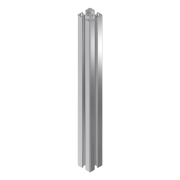
# Autodesk Inventor part: Propile_355
Saved by Autodesk Inventor 2019 (Build 230136000, 136)
## iProperties
Created: 2019-04-24
Part Number: Propile_355
Material: 알루미늄 6061
Document SubType Name: Modeling
Designer: hinmo
Mass: 308.007 g
Surface Area: 1319.64 cm^2
Volume: 114.076 cm^3
Density: 2.7 g/cm^3
Appearance: 알루미늄 - 평지
Author: hinmo
Autodesk Inventor part; units mm, degrees
ref_plane "YZ Plane" through (0, 0, 0) normal (1, 0, 0) x (0, 1, 0)
ref_plane "XZ Plane" through (0, 0, 0) normal (0, 1, 0) x (-1, 0, 0)
ref_plane "XY Plane" through (0, 0, 0) normal (0, 0, 1) x (1, 0, 0)
sketch "스케치1" plane through (0, 0, 0) normal (0, 1, 0) x (-1, 0, 0)
  arc A0 (-198.9025, -155.31) -> (-197.9025, -154.31) centre (-198.9025, -154.31) ccw projected
  line L0 (-197.9025, -154.31) -> (-197.9025, -152.81) projected
  line L1 (-197.9025, -152.81) -> (-199.8525, -152.81) projected
  line L2 (-199.8525, -152.81) -> (-200.8313, -149.1169) projected
  arc A1 (-198.1875, -144.81) -> (-200.8313, -149.1169) centre (-194.1553, -150.25) ccw projected
  line L3 (-198.1875, -144.81) -> (-195.2525, -144.81) projected
  line L4 (-195.2525, -144.81) -> (-194.7525, -144.31) projected
  line L5 (-194.7525, -144.31) -> (-194.2525, -144.81) projected
  line L6 (-194.2525, -144.81) -> (-191.3175, -144.81) projected
  arc A2 (-188.6738, -149.1169) -> (-191.3175, -144.81) centre (-195.3497, -150.25) ccw projected
  line L7 (-188.6738, -149.1169) -> (-189.6525, -152.81) projected
  line L8 (-189.6525, -152.81) -> (-191.6025, -152.81) projected
  line L9 (-191.6025, -152.81) -> (-191.6025, -154.31) projected
  arc A3 (-191.6025, -154.31) -> (-190.6025, -155.31) centre (-190.6025, -154.31) ccw projected
  line L10 (-190.6025, -155.31) -> (-181.2525, -155.31) projected
  arc A4 (-181.2525, -155.31) -> (-179.7525, -153.81) centre (-181.2525, -153.81) ccw projected
  line L11 (-179.7525, -153.81) -> (-179.7525, -144.46) projected
  arc A5 (-179.7525, -144.46) -> (-180.7525, -143.46) centre (-180.7525, -144.46) ccw projected
  line L12 (-180.7525, -143.46) -> (-182.2525, -143.46) projected
  line L13 (-182.2525, -143.46) -> (-182.2525, -145.41) projected
  line L14 (-182.2525, -145.41) -> (-185.9457, -146.3887) projected
  arc A6 (-190.2525, -143.745) -> (-185.9457, -146.3887) centre (-184.8126, -139.7128) ccw projected
  line L15 (-190.2525, -143.745) -> (-190.2525, -140.81) projected
  line L16 (-190.2525, -140.81) -> (-190.7525, -140.31) projected
  line L17 (-190.7525, -140.31) -> (-190.2525, -139.81) projected
  line L18 (-190.2525, -139.81) -> (-190.2525, -136.875) projected
  arc A7 (-185.9457, -134.2313) -> (-190.2525, -136.875) centre (-184.8126, -140.9072) ccw projected
  line L19 (-185.9457, -134.2313) -> (-182.2525, -135.21) projected
  line L20 (-182.2525, -135.21) -> (-182.2525, -137.16) projected
  line L21 (-182.2525, -137.16) -> (-180.7525, -137.16) projected
  arc A8 (-180.7525, -137.16) -> (-179.7525, -136.16) centre (-180.7525, -136.16) ccw projected
  line L22 (-179.7525, -136.16) -> (-179.7525, -126.81) projected
  arc A9 (-179.7525, -126.81) -> (-181.2525, -125.31) centre (-181.2525, -126.81) ccw projected
  line L23 (-181.2525, -125.31) -> (-190.6025, -125.31) projected
  arc A10 (-190.6025, -125.31) -> (-191.6025, -126.31) centre (-190.6025, -126.31) ccw projected
  line L24 (-191.6025, -126.31) -> (-191.6025, -127.81) projected
  line L25 (-191.6025, -127.81) -> (-189.6525, -127.81) projected
  line L26 (-189.6525, -127.81) -> (-188.6738, -131.5032) projected
  arc A11 (-191.3175, -135.81) -> (-188.6738, -131.5032) centre (-195.3497, -130.37) ccw projected
  line L27 (-191.3175, -135.81) -> (-194.2525, -135.81) projected
  line L28 (-194.2525, -135.81) -> (-194.7525, -136.31) projected
  line L29 (-194.7525, -136.31) -> (-195.2525, -135.81) projected
  line L30 (-195.2525, -135.81) -> (-198.1875, -135.81) projected
  arc A12 (-200.8313, -131.5032) -> (-198.1875, -135.81) centre (-194.1553, -130.37) ccw projected
  line L31 (-200.8313, -131.5032) -> (-199.8525, -127.81) projected
  line L32 (-199.8525, -127.81) -> (-197.9025, -127.81) projected
  line L33 (-197.9025, -127.81) -> (-197.9025, -126.31) projected
  arc A13 (-197.9025, -126.31) -> (-198.9025, -125.31) centre (-198.9025, -126.31) ccw projected
  line L34 (-198.9025, -125.31) -> (-208.2525, -125.31) projected
  arc A14 (-208.2525, -125.31) -> (-209.7525, -126.81) centre (-208.2525, -126.81) ccw projected
  line L35 (-209.7525, -126.81) -> (-209.7525, -136.16) projected
  arc A15 (-209.7525, -136.16) -> (-208.7525, -137.16) centre (-208.7525, -136.16) ccw projected
  line L36 (-208.7525, -137.16) -> (-207.2525, -137.16) projected
  line L37 (-207.2525, -137.16) -> (-207.2525, -135.21) projected
  line L38 (-207.2525, -135.21) -> (-203.5594, -134.2313) projected
  arc A16 (-199.2525, -136.875) -> (-203.5594, -134.2313) centre (-204.6925, -140.9072) ccw projected
  line L39 (-199.2525, -136.875) -> (-199.2525, -139.81) projected
  line L40 (-199.2525, -139.81) -> (-198.7525, -140.31) projected
  line L41 (-198.7525, -140.31) -> (-199.2525, -140.81) projected
  line L42 (-199.2525, -140.81) -> (-199.2525, -143.745) projected
  arc A17 (-203.5594, -146.3887) -> (-199.2525, -143.745) centre (-204.6925, -139.7128) ccw projected
  line L43 (-203.5594, -146.3887) -> (-207.2525, -145.41) projected
  line L44 (-207.2525, -145.41) -> (-207.2525, -143.46) projected
  line L45 (-207.2525, -143.46) -> (-208.7525, -143.46) projected
  arc A18 (-208.7525, -143.46) -> (-209.7525, -144.46) centre (-208.7525, -144.46) ccw projected
  line L46 (-209.7525, -144.46) -> (-209.7525, -153.81) projected
  arc A19 (-209.7525, -153.81) -> (-208.2525, -155.31) centre (-208.2525, -153.81) ccw projected
  line L47 (-208.2525, -155.31) -> (-198.9025, -155.31) projected
  arc A20 (-182.1682, -131.8336) -> (-182.1682, -128.7864) centre (-184.7525, -130.31) ccw projected
  line L48 (-182.1682, -131.8336) -> (-181.2222, -132.7797) projected
  line L49 (-181.2222, -132.7797) -> (-182.2829, -133.8403) projected
  line L50 (-182.2829, -133.8403) -> (-183.2289, -132.8943) projected
  arc A21 (-186.2762, -132.8943) -> (-183.2289, -132.8943) centre (-184.7525, -130.31) ccw projected
  line L51 (-186.2762, -132.8943) -> (-187.2222, -133.8403) projected
  line L52 (-187.2222, -133.8403) -> (-188.2829, -132.7797) projected
  line L53 (-188.2829, -132.7797) -> (-187.3368, -131.8336) projected
  arc A22 (-187.3368, -128.7864) -> (-187.3368, -131.8336) centre (-184.7525, -130.31) ccw projected
  line L54 (-187.3368, -128.7864) -> (-188.2829, -127.8403) projected
  line L55 (-188.2829, -127.8403) -> (-187.2222, -126.7797) projected
  line L56 (-187.2222, -126.7797) -> (-186.2762, -127.7257) projected
  arc A23 (-183.2289, -127.7257) -> (-186.2762, -127.7257) centre (-184.7525, -130.31) ccw projected
  line L57 (-183.2289, -127.7257) -> (-182.2829, -126.7797) projected
  line L58 (-182.2829, -126.7797) -> (-181.2222, -127.8403) projected
  line L59 (-181.2222, -127.8403) -> (-182.1682, -128.7864) projected
  line L60 (-191.7222, -138.3403) -> (-192.6564, -138.9476) projected
  arc A24 (-192.6564, -141.6725) -> (-192.6564, -138.9476) centre (-194.7525, -140.31) ccw projected
  line L61 (-192.6564, -141.6725) -> (-191.7222, -142.2797) projected
  line L62 (-191.7222, -142.2797) -> (-192.7829, -143.3403) projected
  line L63 (-192.7829, -143.3403) -> (-193.3901, -142.4061) projected
  arc A25 (-196.115, -142.4061) -> (-193.3901, -142.4061) centre (-194.7525, -140.31) ccw projected
  line L64 (-196.115, -142.4061) -> (-196.7222, -143.3403) projected
  line L65 (-196.7222, -143.3403) -> (-197.7829, -142.2797) projected
  line L66 (-197.7829, -142.2797) -> (-196.8487, -141.6725) projected
  arc A26 (-196.8487, -138.9476) -> (-196.8487, -141.6725) centre (-194.7525, -140.31) ccw projected
  line L67 (-196.8487, -138.9476) -> (-197.7829, -138.3403) projected
  line L68 (-197.7829, -138.3403) -> (-196.7222, -137.2797) projected
  line L69 (-196.7222, -137.2797) -> (-196.115, -138.2139) projected
  arc A27 (-193.3901, -138.2139) -> (-196.115, -138.2139) centre (-194.7525, -140.31) ccw projected
  line L70 (-193.3901, -138.2139) -> (-192.7829, -137.2797) projected
  line L71 (-192.7829, -137.2797) -> (-191.7222, -138.3403) projected
  arc A28 (-183.2289, -147.7257) -> (-186.2762, -147.7257) centre (-184.7525, -150.31) ccw projected
  line L72 (-183.2289, -147.7257) -> (-182.2829, -146.7797) projected
  line L73 (-182.2829, -146.7797) -> (-181.2222, -147.8403) projected
  line L74 (-181.2222, -147.8403) -> (-182.1682, -148.7864) projected
  arc A29 (-182.1682, -151.8336) -> (-182.1682, -148.7864) centre (-184.7525, -150.31) ccw projected
  line L75 (-182.1682, -151.8336) -> (-181.2222, -152.7797) projected
  line L76 (-181.2222, -152.7797) -> (-182.2829, -153.8403) projected
  line L77 (-182.2829, -153.8403) -> (-183.2289, -152.8943) projected
  arc A30 (-186.2762, -152.8943) -> (-183.2289, -152.8943) centre (-184.7525, -150.31) ccw projected
  line L78 (-186.2762, -152.8943) -> (-187.2222, -153.8403) projected
  line L79 (-187.2222, -153.8403) -> (-188.2829, -152.7797) projected
  line L80 (-188.2829, -152.7797) -> (-187.3368, -151.8336) projected
  arc A31 (-187.3368, -148.7864) -> (-187.3368, -151.8336) centre (-184.7525, -150.31) ccw projected
  line L81 (-187.3368, -148.7864) -> (-188.2829, -147.8403) projected
  line L82 (-188.2829, -147.8403) -> (-187.2222, -146.7797) projected
  line L83 (-187.2222, -146.7797) -> (-186.2762, -147.7257) projected
  arc A32 (-206.2762, -132.8943) -> (-203.2289, -132.8943) centre (-204.7525, -130.31) ccw projected
  line L84 (-206.2762, -132.8943) -> (-207.2222, -133.8403) projected
  line L85 (-207.2222, -133.8403) -> (-208.2829, -132.7797) projected
  line L86 (-208.2829, -132.7797) -> (-207.3368, -131.8336) projected
  arc A33 (-207.3368, -128.7864) -> (-207.3368, -131.8336) centre (-204.7525, -130.31) ccw projected
  line L87 (-207.3368, -128.7864) -> (-208.2829, -127.8403) projected
  line L88 (-208.2829, -127.8403) -> (-207.2222, -126.7797) projected
  line L89 (-207.2222, -126.7797) -> (-206.2762, -127.7257) projected
  arc A34 (-203.2289, -127.7257) -> (-206.2762, -127.7257) centre (-204.7525, -130.31) ccw projected
  line L90 (-203.2289, -127.7257) -> (-202.2829, -126.7797) projected
  line L91 (-202.2829, -126.7797) -> (-201.2222, -127.8403) projected
  line L92 (-201.2222, -127.8403) -> (-202.1682, -128.7864) projected
  arc A35 (-202.1682, -131.8336) -> (-202.1682, -128.7864) centre (-204.7525, -130.31) ccw projected
  line L93 (-202.1682, -131.8336) -> (-201.2222, -132.7797) projected
  line L94 (-201.2222, -132.7797) -> (-202.2829, -133.8403) projected
  line L95 (-202.2829, -133.8403) -> (-203.2289, -132.8943) projected
  arc A36 (-202.1682, -151.8336) -> (-202.1682, -148.7864) centre (-204.7525, -150.31) ccw projected
  line L96 (-202.1682, -151.8336) -> (-201.2222, -152.7797) projected
  line L97 (-201.2222, -152.7797) -> (-202.2829, -153.8403) projected
  line L98 (-202.2829, -153.8403) -> (-203.2289, -152.8943) projected
  arc A37 (-206.2762, -152.8943) -> (-203.2289, -152.8943) centre (-204.7525, -150.31) ccw projected
  line L99 (-206.2762, -152.8943) -> (-207.2222, -153.8403) projected
  line L100 (-207.2222, -153.8403) -> (-208.2829, -152.7797) projected
  line L101 (-208.2829, -152.7797) -> (-207.3368, -151.8336) projected
  arc A38 (-207.3368, -148.7864) -> (-207.3368, -151.8336) centre (-204.7525, -150.31) ccw projected
  line L102 (-207.3368, -148.7864) -> (-208.2829, -147.8403) projected
  line L103 (-208.2829, -147.8403) -> (-207.2222, -146.7797) projected
  line L104 (-207.2222, -146.7797) -> (-206.2762, -147.7257) projected
  arc A39 (-203.2289, -147.7257) -> (-206.2762, -147.7257) centre (-204.7525, -150.31) ccw projected
  line L105 (-203.2289, -147.7257) -> (-202.2829, -146.7797) projected
  line L106 (-202.2829, -146.7797) -> (-201.2222, -147.8403) projected
  line L107 (-201.2222, -147.8403) -> (-202.1682, -148.7864) projected
  arc A40 (-4.15, -15) -> (-3.15, -14) centre (-4.15, -14) ccw
  line L108 (-3.15, -14) -> (-3.15, -12.5)
  line L109 (-3.15, -12.5) -> (-5.1, -12.5)
  line L110 (-5.1, -12.5) -> (-6.0787, -8.8068)
  arc A41 (-3.435, -4.5) -> (-6.0787, -8.8068) centre (0.5972, -9.94) ccw
  line L111 (-3.435, -4.5) -> (-0.5, -4.5)
  line L112 (-0.5, -4.5) -> (0, -4)
  line L113 (0, -4) -> (0.5, -4.5)
  line L114 (0.5, -4.5) -> (3.435, -4.5)
  arc A42 (6.0787, -8.8068) -> (3.435, -4.5) centre (-0.5972, -9.94) ccw
  line L115 (6.0787, -8.8068) -> (5.1, -12.5)
  line L116 (5.1, -12.5) -> (3.15, -12.5)
  line L117 (3.15, -12.5) -> (3.15, -14)
  arc A43 (3.15, -14) -> (4.15, -15) centre (4.15, -14) ccw
  line L118 (4.15, -15) -> (13.5, -15)
  arc A44 (13.5, -15) -> (15, -13.5) centre (13.5, -13.5) ccw
  line L119 (15, -13.5) -> (15, -4.15)
  arc A45 (15, -4.15) -> (14, -3.15) centre (14, -4.15) ccw
  line L120 (14, -3.15) -> (12.5, -3.15)
  line L121 (12.5, -3.15) -> (12.5, -5.1)
  line L122 (12.5, -5.1) -> (8.8068, -6.0787)
  arc A46 (4.5, -3.435) -> (8.8068, -6.0787) centre (9.94, 0.5972) ccw
  line L123 (4.5, -3.435) -> (4.5, -0.5)
  line L124 (4.5, -0.5) -> (4, 0)
  line L125 (4, 0) -> (4.5, 0.5)
  line L126 (4.5, 0.5) -> (4.5, 3.435)
  arc A47 (8.8068, 6.0787) -> (4.5, 3.435) centre (9.94, -0.5972) ccw
  line L127 (8.8068, 6.0787) -> (12.5, 5.1)
  line L128 (12.5, 5.1) -> (12.5, 3.15)
  line L129 (12.5, 3.15) -> (14, 3.15)
  arc A48 (14, 3.15) -> (15, 4.15) centre (14, 4.15) ccw
  line L130 (15, 4.15) -> (15, 13.5)
  arc A49 (15, 13.5) -> (13.5, 15) centre (13.5, 13.5) ccw
  line L131 (13.5, 15) -> (4.15, 15)
  arc A50 (4.15, 15) -> (3.15, 14) centre (4.15, 14) ccw
  line L132 (3.15, 14) -> (3.15, 12.5)
  line L133 (3.15, 12.5) -> (5.1, 12.5)
  line L134 (5.1, 12.5) -> (6.0787, 8.8068)
  arc A51 (3.435, 4.5) -> (6.0787, 8.8068) centre (-0.5972, 9.94) ccw
  line L135 (3.435, 4.5) -> (0.5, 4.5)
  line L136 (0.5, 4.5) -> (0, 4)
  line L137 (0, 4) -> (-0.5, 4.5)
  line L138 (-0.5, 4.5) -> (-3.435, 4.5)
  arc A52 (-6.0787, 8.8068) -> (-3.435, 4.5) centre (0.5972, 9.94) ccw
  line L139 (-6.0787, 8.8068) -> (-5.1, 12.5)
  line L140 (-5.1, 12.5) -> (-3.15, 12.5)
  line L141 (-3.15, 12.5) -> (-3.15, 14)
  arc A53 (-3.15, 14) -> (-4.15, 15) centre (-4.15, 14) ccw
  line L142 (-4.15, 15) -> (-13.5, 15)
  arc A54 (-13.5, 15) -> (-15, 13.5) centre (-13.5, 13.5) ccw
  line L143 (-15, 13.5) -> (-15, 4.15)
  arc A55 (-15, 4.15) -> (-14, 3.15) centre (-14, 4.15) ccw
  line L144 (-14, 3.15) -> (-12.5, 3.15)
  line L145 (-12.5, 3.15) -> (-12.5, 5.1)
  line L146 (-12.5, 5.1) -> (-8.8068, 6.0787)
  arc A56 (-4.5, 3.435) -> (-8.8068, 6.0787) centre (-9.94, -0.5972) ccw
  line L147 (-4.5, 3.435) -> (-4.5, 0.5)
  line L148 (-4.5, 0.5) -> (-4, 0)
  line L149 (-4, 0) -> (-4.5, -0.5)
  line L150 (-4.5, -0.5) -> (-4.5, -3.435)
  arc A57 (-8.8068, -6.0787) -> (-4.5, -3.435) centre (-9.94, 0.5972) ccw
  line L151 (-8.8068, -6.0787) -> (-12.5, -5.1)
  line L152 (-12.5, -5.1) -> (-12.5, -3.15)
  line L153 (-12.5, -3.15) -> (-14, -3.15)
  arc A58 (-14, -3.15) -> (-15, -4.15) centre (-14, -4.15) ccw
  line L154 (-15, -4.15) -> (-15, -13.5)
  arc A59 (-15, -13.5) -> (-13.5, -15) centre (-13.5, -13.5) ccw
  line L155 (-13.5, -15) -> (-4.15, -15)
  arc A60 (12.5843, 8.4764) -> (12.5843, 11.5236) centre (10, 10) ccw
  line L156 (12.5843, 8.4764) -> (13.5303, 7.5303)
  line L157 (13.5303, 7.5303) -> (12.4697, 6.4697)
  line L158 (12.4697, 6.4697) -> (11.5236, 7.4157)
  arc A61 (8.4764, 7.4157) -> (11.5236, 7.4157) centre (10, 10) ccw
  line L159 (8.4764, 7.4157) -> (7.5303, 6.4697)
  line L160 (7.5303, 6.4697) -> (6.4697, 7.5303)
  line L161 (6.4697, 7.5303) -> (7.4157, 8.4764)
  arc A62 (7.4157, 11.5236) -> (7.4157, 8.4764) centre (10, 10) ccw
  line L162 (7.4157, 11.5236) -> (6.4697, 12.4697)
  line L163 (6.4697, 12.4697) -> (7.5303, 13.5303)
  line L164 (7.5303, 13.5303) -> (8.4764, 12.5843)
  arc A63 (11.5236, 12.5843) -> (8.4764, 12.5843) centre (10, 10) ccw
  line L165 (11.5236, 12.5843) -> (12.4697, 13.5303)
  line L166 (12.4697, 13.5303) -> (13.5303, 12.4697)
  line L167 (13.5303, 12.4697) -> (12.5843, 11.5236)
  line L168 (3.0303, 1.9697) -> (2.0961, 1.3624)
  arc A64 (2.0961, -1.3624) -> (2.0961, 1.3624) centre (0, 0) ccw
  line L169 (2.0961, -1.3624) -> (3.0303, -1.9697)
  line L170 (3.0303, -1.9697) -> (1.9697, -3.0303)
  line L171 (1.9697, -3.0303) -> (1.3624, -2.0961)
  arc A65 (-1.3624, -2.0961) -> (1.3624, -2.0961) centre (0, 0) ccw
  line L172 (-1.3624, -2.0961) -> (-1.9697, -3.0303)
  line L173 (-1.9697, -3.0303) -> (-3.0303, -1.9697)
  line L174 (-3.0303, -1.9697) -> (-2.0961, -1.3624)
  arc A66 (-2.0961, 1.3624) -> (-2.0961, -1.3624) centre (0, 0) ccw
  line L175 (-2.0961, 1.3624) -> (-3.0303, 1.9697)
  line L176 (-3.0303, 1.9697) -> (-1.9697, 3.0303)
  line L177 (-1.9697, 3.0303) -> (-1.3624, 2.0961)
  arc A67 (1.3624, 2.0961) -> (-1.3624, 2.0961) centre (0, 0) ccw
  line L178 (1.3624, 2.0961) -> (1.9697, 3.0303)
  line L179 (1.9697, 3.0303) -> (3.0303, 1.9697)
  arc A68 (11.5236, -7.4157) -> (8.4764, -7.4157) centre (10, -10) ccw
  line L180 (11.5236, -7.4157) -> (12.4697, -6.4697)
  line L181 (12.4697, -6.4697) -> (13.5303, -7.5303)
  line L182 (13.5303, -7.5303) -> (12.5843, -8.4764)
  arc A69 (12.5843, -11.5236) -> (12.5843, -8.4764) centre (10, -10) ccw
  line L183 (12.5843, -11.5236) -> (13.5303, -12.4697)
  line L184 (13.5303, -12.4697) -> (12.4697, -13.5303)
  line L185 (12.4697, -13.5303) -> (11.5236, -12.5843)
  arc A70 (8.4764, -12.5843) -> (11.5236, -12.5843) centre (10, -10) ccw
  line L186 (8.4764, -12.5843) -> (7.5303, -13.5303)
  line L187 (7.5303, -13.5303) -> (6.4697, -12.4697)
  line L188 (6.4697, -12.4697) -> (7.4157, -11.5236)
  arc A71 (7.4157, -8.4764) -> (7.4157, -11.5236) centre (10, -10) ccw
  line L189 (7.4157, -8.4764) -> (6.4697, -7.5303)
  line L190 (6.4697, -7.5303) -> (7.5303, -6.4697)
  line L191 (7.5303, -6.4697) -> (8.4764, -7.4157)
  arc A72 (-11.5236, 7.4157) -> (-8.4764, 7.4157) centre (-10, 10) ccw
  line L192 (-11.5236, 7.4157) -> (-12.4697, 6.4697)
  line L193 (-12.4697, 6.4697) -> (-13.5303, 7.5303)
  line L194 (-13.5303, 7.5303) -> (-12.5843, 8.4764)
  arc A73 (-12.5843, 11.5236) -> (-12.5843, 8.4764) centre (-10, 10) ccw
  line L195 (-12.5843, 11.5236) -> (-13.5303, 12.4697)
  line L196 (-13.5303, 12.4697) -> (-12.4697, 13.5303)
  line L197 (-12.4697, 13.5303) -> (-11.5236, 12.5843)
  arc A74 (-8.4764, 12.5843) -> (-11.5236, 12.5843) centre (-10, 10) ccw
  line L198 (-8.4764, 12.5843) -> (-7.5303, 13.5303)
  line L199 (-7.5303, 13.5303) -> (-6.4697, 12.4697)
  line L200 (-6.4697, 12.4697) -> (-7.4157, 11.5236)
  arc A75 (-7.4157, 8.4764) -> (-7.4157, 11.5236) centre (-10, 10) ccw
  line L201 (-7.4157, 8.4764) -> (-6.4697, 7.5303)
  line L202 (-6.4697, 7.5303) -> (-7.5303, 6.4697)
  line L203 (-7.5303, 6.4697) -> (-8.4764, 7.4157)
  arc A76 (-7.4157, -11.5236) -> (-7.4157, -8.4764) centre (-10, -10) ccw
  line L204 (-7.4157, -11.5236) -> (-6.4697, -12.4697)
  line L205 (-6.4697, -12.4697) -> (-7.5303, -13.5303)
  line L206 (-7.5303, -13.5303) -> (-8.4764, -12.5843)
  arc A77 (-11.5236, -12.5843) -> (-8.4764, -12.5843) centre (-10, -10) ccw
  line L207 (-11.5236, -12.5843) -> (-12.4697, -13.5303)
  line L208 (-12.4697, -13.5303) -> (-13.5303, -12.4697)
  line L209 (-13.5303, -12.4697) -> (-12.5843, -11.5236)
  arc A78 (-12.5843, -8.4764) -> (-12.5843, -11.5236) centre (-10, -10) ccw
  line L210 (-12.5843, -8.4764) -> (-13.5303, -7.5303)
  line L211 (-13.5303, -7.5303) -> (-12.4697, -6.4697)
  line L212 (-12.4697, -6.4697) -> (-11.5236, -7.4157)
  arc A79 (-8.4764, -7.4157) -> (-11.5236, -7.4157) centre (-10, -10) ccw
  line L213 (-8.4764, -7.4157) -> (-7.5303, -6.4697)
  line L214 (-7.5303, -6.4697) -> (-6.4697, -7.5303)
  line L215 (-6.4697, -7.5303) -> (-7.4157, -8.4764)
  constraints: 216 end point, 80 point on circle, 40 centre point
extrude "돌출1" add sketch "스케치1" along normal blind 305 contours L155 A59 L154 A58 L153 L152 L151 A57 L150 L149 L148 L147 A56 L146 L145 L144 A55 L143 A54 L142 A53 L141 L140 L139 A52 L138 L137 L136 L135 A51 L134 L133 L132 A50 L131 A49 L130 A48 L129 L128 L127 A47 L126 L125 L124 L123 A46 L122 L121 L120 A45 L119 A44 L118 A43 L117 L116 L115 A42 L114 L113 L112 L111 A41 L110 L109 L108 A40
